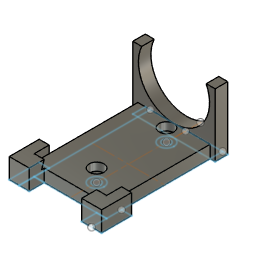
CV60 Camera Holder 2.0 v9 (Autodesk Fusion 360 design; units mm, degrees)
Autodesk Fusion 360 part; units mm, degrees
sketch "Schizzo1" plane through (0, 0, 0) normal (0, 0, 1) x (1, 0, 0)
  line L0 (-339.0462, -7.6484) -> (-310.0462, -7.6484)
  line L1 (-310.0462, -7.6484) -> (-310.0462, 38.8516)
  line L2 (-339.0462, 38.8516) -> (-339.0462, -7.6484)
  line L3 (-324.5462, 38.8516) -> (-324.5462, -7.6484)
  line L4 (-339.0462, 15.6016) -> (-310.0462, 15.6016)
  line L5 (-308.0462, 38.8516) -> (-308.0462, 33.8516)
  line L6 (-308.0462, 33.8516) -> (-341.0462, 33.8516)
  line L7 (-341.0462, 33.8516) -> (-341.0462, 38.8516)
  line L8 (-324.5462, 38.8516) -> (-324.5462, 33.8516)
  line L9 (-339.0462, -7.6484) -> (-335.0462, -7.6484)
  line L10 (-335.0462, -7.6484) -> (-335.0462, -13.6484)
  line L11 (-335.0462, -13.6484) -> (-339.0462, -13.6484)
  line L12 (-339.0462, -13.6484) -> (-339.0462, -7.6484)
  line L13 (-310.0462, -13.6484) -> (-310.0462, -7.6484)
  line L14 (-314.0462, -7.6484) -> (-314.0462, -13.6484)
  line L15 (-314.0462, -13.6484) -> (-310.0462, -13.6484)
  line L16 (-310.0462, -7.6484) -> (-314.0462, -7.6484)
  line L17 (-339.0462, 33.8516) -> (-308.0462, 33.8516) construction
  line L18 (-308.0462, 38.8516) -> (-341.0462, 38.8516)
  line L19 (-324.5462, 44.5) -> (-324.5462, 38.5) construction
  circle A0 centre (-324.5462, 30.8516) radius 1.6
  circle A1 centre (-324.5462, 2.8516) radius 1.6
  circle A2 centre (-324.5462, 2.8516) radius 2.95
  circle A3 centre (-324.5462, 30.8516) radius 2.95
  line L20 (-339.0462, -13.6484) -> (-343.0462, -13.6484)
  line L21 (-343.0462, -13.6484) -> (-343.0462, -1.6484)
  line L22 (-343.0462, -1.6484) -> (-339.0462, -1.6484)
  line L23 (-339.0462, -1.6484) -> (-339.0462, -13.6484)
  line L24 (-306.0462, -1.6484) -> (-310.0462, -1.6484)
  line L25 (-306.0462, -13.6484) -> (-306.0462, -1.6484)
  line L26 (-310.0462, -13.6484) -> (-306.0462, -13.6484)
  dimension "d420" = 29
  dimension "d422" = 33
  dimension "d423" = 5
  dimension "d442" = 4
  dimension "d443" = 6
  dimension "d640" = 3.2
  dimension "d641" = 3.2
  dimension "d642" = 28
  dimension "d643" = 5.9
  dimension "d644" = 5.9
  dimension "d648" = 8
  dimension "d652" = 4
  dimension "d653" = 12
  dimension "d658" = 46.5
  dimension "d665" = 37
  constraint horizontal L0
  constraint vertical L1
  constraint vertical L2
  constraint midpoint L0 L3.end
  constraint midpoint L2 L4.start
  constraint midpoint L1 L4.end
  constraint vertical L5
  constraint horizontal L6
  constraint vertical L7
  constraint midpoint L6 L8.end
  constraint coincident L3.start L8.start
  constraint horizontal L9
  constraint vertical L10
  constraint horizontal L11
  constraint vertical L12
  constraint symmetric L0.start L3 L0.end
  constraint symmetric L3 L9.end L14.start
  constraint symmetric L3 L10.end L14.end
  constraint symmetric L3 L11.end L13.start
  constraint coincident L6 L17.start
  constraint coincident L2 L17.start
  constraint perpendicular L2 L17
  constraint perpendicular L7 L18
  constraint coincident L3 A0.centre
  constraint coincident L3 A1.centre
  constraint concentric A1 A2
  constraint concentric A0 A3
  constraint horizontal L20
  constraint vertical L21
  constraint horizontal L22
  constraint vertical L23
  constraint symmetric L3 L20.end L25.start
  constraint symmetric L3 L21.end L24.start
  constraint symmetric L3 L22.end L24.end
  measures "d420" distance of L0.start L0.end
  measures "d422" distance of L7.end L5.start
  measures "d423" distance of L7.end L6.end
  measures "d442" distance of L0.start L9.end
  measures "d443" distance of L0.start L11.end
  measures "d640" diameter of A0
  measures "d641" diameter of A1
  measures "d642" distance of A0.centre A1.centre
  measures "d643" diameter of A2
  measures "d644" diameter of A3
  measures "d648" distance of L18 A0.centre
  measures "d652" distance of L11.end L20.end
  measures "d653" distance of L11.end L22.end
  measures "d658" distance of L0 L18
  measures "d665" distance of L21 L25
extrude "Estrusione97" add sketch "Schizzo1" along normal blind 5 contours L0 L2 L3 L4 L9 A2 L23 | L0 L1 L3 L4 L16 A2 | L2 L3 L4 L6 A3 | L3 A1 A2 | L3 A1 A2 | L2 L6 L7 L18 | L2 L3 L6 L8 L18 | L1 L3 L4 L6 A3 | L1 L3 L6 L8 L18 | L3 A0 A3 | L3 A0 A3 | L1 L5 L6 L18
extrude "Estrusione140" cut sketch "Schizzo1" against normal blind 3.2 from surface at 5 contours L3 A1 A2 | L3 A1 A2 | L3 A0 A3 | L3 A0 A3
extrude "Estrusione98" add sketch "Schizzo1" along normal up to surface (33.5 mm away) contours L2 L6 L7 L18 | L2 L3 L6 L8 L18 | L1 L3 L6 L8 L18 | L1 L5 L6 L18
extrude "Estrusione102" add sketch "Schizzo1" along normal up to surface (8 mm away) contours L0 L9 L10 L11 L12 L23 | L0 L13 L14 L15 L16
sketch "Schizzo45" plane through (0, 38.8516, 0) normal (0, 1, 0) x (-1, 0, 0)
  line L0 (341.0462, 0) -> (341.0462, 33.5)
  line L1 (308.0462, 33.5) -> (308.0462, 0)
  line L2 (308.0462, 0) -> (341.0462, 0)
  line L3 (308.0462, 33.5) -> (341.0462, 33.5) construction
  line L4 (341.0462, 33.5) -> (341.0462, 1.9118) construction
  line L5 (341.0462, 1.9118) -> (308.0462, 1.9118) construction
  line L6 (308.0462, 1.9118) -> (308.0462, 33.5) construction
  line L7 (308.0462, 17.7059) -> (341.0462, 17.7059) construction
  circle A0 centre (324.5462, 19.25) radius 14.25
  line L8 (308.0462, 25.25) -> (341.0462, 25.25)
  line L9 (308.0462, 0) -> (341.0462, 0)
  line L10 (324.5462, 0) -> (324.5462, 36.5) construction
  line L11 (341.0462, 33.5) -> (308.0462, 33.5)
  dimension "d560" = 28.5
  dimension "d561" = 6
  dimension "d584" = 19.25
  constraint horizontal L3
  constraint vertical L4
  constraint horizontal L5
  constraint vertical L6
  constraint midpoint L6 L7.start
  constraint midpoint L4 L7.end
  constraint coincident L1 L8.start
  constraint coincident L4 L8.end
  constraint perpendicular L4 L8
  constraint midpoint L9 L10.start
  constraint coincident A0.centre L10
  constraint collinear L3 L11
  measures "d560" diameter of A0
  measures "d561" distance of A0.centre L8
  measures "d584" distance of A0.centre L9
extrude "Estrusione128" cut sketch "Schizzo45" against normal blind 7 contours A0 L8 | A0 L8
extrude "Estrusione139" cut sketch "Schizzo45" against normal blind 5 contours L0 A0 L8 L11 | L1 A0 L8 L11
sketch "Schizzo40" plane through (-310.0462, 0, 0) normal (1, 0, 0) x (0, 1, 0)
  line L0 (-13.6484, 0) -> (33.8516, 0)
  line L1 (33.8516, 5) -> (-7.6484, 5)
  line L2 (-7.6484, 8) -> (-13.6484, 8)
  line L3 (-13.6484, 8) -> (-13.6484, 0)
  line L4 (-13.6484, 8) -> (-7.6484, 8) construction
  line L5 (-7.6484, 8) -> (-7.6484, 5) construction
  line L6 (-7.6484, 5) -> (-13.6484, 5) construction
  line L7 (-13.6484, 5) -> (-13.6484, 8) construction
  line L8 (-8.6484, 8) -> (-8.6484, 5) construction
  line L9 (-7.6484, 8) -> (-8.6484, 5)
  line L10 (-8.6484, 5) -> (-7.6484, 5)
  line L11 (-7.6484, 5) -> (-7.6484, 8)
  dimension "d651" = 1
  constraint horizontal L4
  constraint vertical L5
  constraint horizontal L6
  constraint vertical L7
  constraint coincident L2.end L3.start
  constraint coincident L1.end L5.end
  constraint coincident L4 L8.start
  constraint coincident L6 L8.end
  constraint perpendicular L6 L8
  constraint coincident L2.start L4.end
  measures "d651" distance of L5 L8
extrude "Estrusione103" cut sketch "Schizzo40" against normal blind 30
extrude "Estrusione141" add sketch "Schizzo1" along normal blind 8 contours L2 L12 L20 L21 L22 L23 | L1 L13 L24 L25 L26
equation "BeamLenght = 140 mm"
equation "BeamSlotDepth = 16.5 mm"
equation "CableBoreSize = 4 mm"
equation "RotationJontDiameter = 10 mm"
equation "BeamScrewHole = 4 mm"
equation "BeamLock = 8.2 mm"
equation "JointLockDepth = 1 mm"
equation "JointLockStep = 0.5 mm" comment "This is the step before the joint lock sink"
equation "d584 = 5 mm + ( 28.50 / 2 ) * 1 mm"
named bodies: "Camera Holder"
